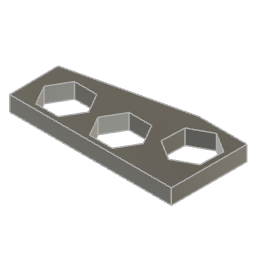
_test_nuts_nyloc.abe879d1-8173-4fa7-98a8-54e223176166 (Autodesk Fusion 360 design; units mm, degrees)
Autodesk Fusion 360 part; units mm, degrees
sketch "Sketch1" plane through (0, 0, 0) normal (0, 0, 1) x (1, 0, 0)
  line L0 (-11.4356, -3.2382) -> (9.9345, -3.2382)
  line L1 (9.9345, -3.2382) -> (9.9345, 6.7515)
  line L2 (-8.6382, 2.5386) -> (-10.1105, -0.0114)
  line L3 (-10.1105, -0.0114) -> (-8.6382, -2.5614)
  line L4 (-8.6382, -2.5614) -> (-5.6937, -2.5614)
  line L5 (-5.6937, -2.5614) -> (-4.2215, -0.0114)
  line L6 (-4.2215, -0.0114) -> (-5.6937, 2.5386)
  line L7 (-5.6937, 2.5386) -> (-8.6382, 2.5386)
  line L8 (6.4738, -0.1404) -> (9.1725, 1.3019)
  line L9 (9.1725, 1.3019) -> (9.2728, 4.3602)
  line L10 (9.2728, 4.3602) -> (6.6744, 5.9762)
  line L11 (6.6744, 5.9762) -> (3.9757, 4.5339)
  line L12 (3.9757, 4.5339) -> (3.8754, 1.4756)
  line L13 (3.8754, 1.4756) -> (6.4738, -0.1404)
  line L14 (3.0022, 0) -> (1.5011, 2.6)
  line L15 (1.5011, 2.6) -> (-1.5011, 2.6)
  line L16 (-1.5011, 2.6) -> (-3.0022, 0)
  line L17 (-3.0022, 0) -> (-1.5011, -2.6)
  line L18 (-1.5011, -2.6) -> (1.5011, -2.6)
  line L19 (1.5011, -2.6) -> (3.0022, 0)
  line L20 (9.9345, 6.7515) -> (3.5648, 6.7515)
  line L21 (3.5648, 6.7515) -> (-11.5106, 3.238)
  line L22 (-11.5106, 3.238) -> (-11.4356, -3.2382)
  point P0 (-7.166, -0.0114)
  point P1 (6.5741, 2.9179)
  constraint horizontal L0
  constraint vertical L1
  constraint perpendicular L1 L20
  measures "d1" distance of L4 L7
  measures "d42" distance of L15 L18
  measures "d43" distance of L9 L12
derive "ExternalDerived1" from "MasterParameters_Gripper v73"
extrude "Extrude1" add sketch "Sketch1" along normal blind 2
equation "d1 = m25_nyloc_width_Ref"
equation "m2_nut_diameter_Ref = 4.2 mm"
equation "m2_nut_height_Ref = 3 mm"
equation "arm_screw_wall_thickness_Ref = 1 mm"
equation "m2_screw_diameter_Ref = 2.2 mm" comment "diameter with tolerance"
equation "m25_screw_diameter_Ref = 2.7 mm"
equation "m25_wall_thickness_Ref = 2 mm"
equation "m2_tapping_tolerance_Ref = 0.2 mm"
equation "Servo_cut_gap_Ref = 0.5 mm"
equation "m25_screw_head_height_Ref = 2.5 mm"
equation "m25_screw_head_width_Ref = 4.6 mm"
equation "m25_arm_screw_plus_tolerance_Ref = 2.9 mm" comment "Additional parameter to experiment with parameter to hopefully enable free movement of arm"
equation "m2_tapping_head_width_Ref = 4.4 mm"
equation "back_arms_thickness_Ref = 8.5 mm"
equation "m2_screw_head_diameter_Ref = 4 mm"
equation "m2_screw_head_height_Ref = 2 mm"
equation "arm_height_Ref = 4 mm"
equation "arm_ground_clearance_Ref = 1 mm"
equation "m3_screw_diameter_Ref = 3.2 mm"
equation "m3_wall_thickness_gripper_mount_Ref = 2 mm"
equation "arm_length_Ref = 27.5 mm"
equation "gear_arm_gap_Ref = 0.05 mm"
equation "distance_lower_upper_plate_Ref = 10 mm"
equation "gear_screw_dist_Ref = 1.5 mm"
equation "gear_z_height_placement_on_arm_Ref = 5 mm"
equation "plate_distance_back_axes_Ref = 30 mm" comment "Distance between back-axes, namely servo and the arm axis of the arm in the back"
equation "distance_arms_front_Ref = 12 mm" comment "Distance from the back to the front axis"
equation "gear_arm_connector_height_Ref = 4 mm"
equation "m25_ruthex_outer_Ref = 7.2 mm"
equation "m25_ruthex_inner_Ref = 4 mm"
equation "m25_ruthex_height_Ref = 5.7 mm"
equation "plate_single_height_Ref = 3 mm" comment "height of a single plate piece"
equation "plate_distance_back_front_y_Ref = 22 mm"
equation "stand_width_Ref = 5 mm" comment "width of the stand that the gripper can be mounted onto"
equation "gripper_tpu_thickness_Ref = 6 mm"
equation "arm_top_tolerance_Ref = 0.2 mm"
equation "gear_square_length_Ref = 5.9 mm"
equation "m25_nyloc_width_Ref = 5.1 mm"
equation "m25_nyloc_height_Ref = 3.8 mm"
equation "d42 = m25_nyloc_width_Ref + 0.1 mm"
equation "d43 = m25_nyloc_width_Ref + 0.2 mm"
